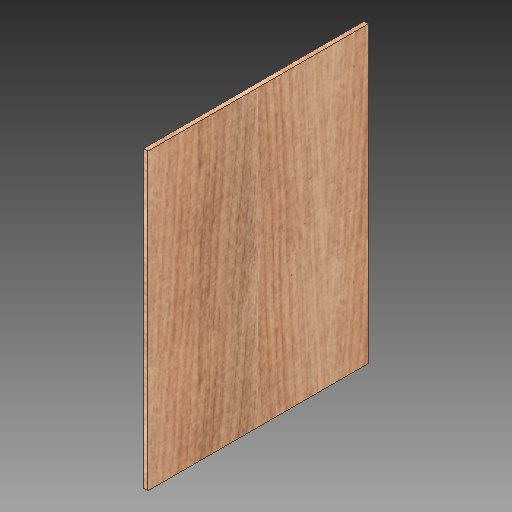
# Autodesk Inventor part: planche_gauche
Saved by Autodesk Inventor 2019 (Build 230136000, 136)
## iProperties
Created: 2018-12-03
Part Number: planche_gauche
Material: Wood (Birch)
Document SubType Name: Modeling
Designer: Bienvenue
Density: 0.55 g/cm^3
Appearance: Birch - Natural Polished
Author: Bienvenue
Autodesk Inventor part; units mm, degrees
ref_plane "YZ Plane" through (0, 0, 0) normal (1, 0, 0) x (0, 1, 0)
ref_plane "XZ Plane" through (0, 0, 0) normal (0, 1, 0) x (-1, 0, 0)
ref_plane "XY Plane" through (0, 0, 0) normal (0, 0, 1) x (1, 0, 0)
sketch "Sketch1" plane through (0, 0, 0) normal (1, 0, 0) x (0, 1, 0)
  line L0 (0, 0) -> (406, 0)
  line L1 (406, 0) -> (406, -300)
  line L2 (406, -300) -> (0, -300)
  line L3 (0, -300) -> (0, 0)
  dimension "d0" = 300
  dimension "d1" = 406
  constraints: 8 end point, 2 parallel, 1 horizontal, 1 perpendicular
  measures "d0" distance of L2.end L0.start
  measures "d1" distance of L0.start L0.end
extrude "Extrusion1" add sketch "Sketch1" along normal blind 6
sketch "Sketch2" plane through (6, 0, 0) normal (1, 0, 0) x (0, 0, -1)
  line L0 (0, 0) -> (300, 0) projected
  line L1 (0, 400) -> (300, 400)
  line L2 (300, 400) -> (300, 0)
  line L3 (300, 0) -> (0, 0)
  line L4 (0, 0) -> (0, 400)
  line L5 (0, 406) -> (0, 0) projected
  line L6 (0, 406) -> (300, 406)
  line L7 (300, 406) -> (300, 400)
  line L8 (300, 400) -> (0, 400)
  line L9 (0, 400) -> (0, 406)
  dimension "d4" = 400
  dimension "d5" = 300
  constraints: 16 end point, 4 parallel, 2 horizontal, 2 perpendicular
  measures "d4" distance of L3.end L1.start
  measures "d5" distance of L1.start L1.end
extrude "Extrusion2" cut sketch "Sketch2" against normal blind 6 contours L5 L6 L7 L1
body "Solid1"
